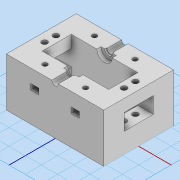
# Autodesk Inventor part: 19_Base_Pezzo_Unico
Saved by Autodesk Inventor 2020 (Build 240168000, 168)
## iProperties
Created: 2019-10-24
Part Number: 19_Base_Pezzo_Unico
Material: Generico
Document SubType Name: Modeling
Designer: socci
Density: 1 g/cm^3
Appearance: Default
Author: socci
Autodesk Inventor part; units mm, degrees
ref_plane "YZ Plane" through (0, 0, 0) normal (1, 0, 0) x (0, 1, 0)
ref_plane "XZ Plane" through (0, 0, 0) normal (0, 1, 0) x (-1, 0, 0)
ref_plane "XY Plane" through (0, 0, 0) normal (0, 0, 1) x (1, 0, 0)
sketch "Schizzo1" plane through (0, 0, 0) normal (0, 1, 0) x (-1, 0, 0)
  line L0 (60, 43) -> (-60, 43)
  line L1 (-60, 43) -> (-60, -43)
  line L2 (-60, -43) -> (60, -43)
  line L3 (60, -43) -> (60, 43)
  line L4 (60, 43) -> (-60, -43) construction
  line L5 (-60, 43) -> (60, -43) construction
  point P0 (0, 0)
  point P1 (0, 0)
  point P2 (0, 0)
  dimension "d0" = 120
  dimension "d1" = 86
  constraints: 12 end point, 3 midpoint, 2 parallel, 1 coincident, 1 horizontal, 1 perpendicular
  measures "d0" distance of L0.start L0.end
  measures "d1" distance of L2.end L0.start
extrude "Estrusione1" add sketch "Schizzo1" along normal blind 60
sketch "Schizzo2" plane through (60, 0, 43) normal (1, 0, 0) x (0, 0, -1)
  line L0 (43, 0) -> (43, 15)
  line L1 (25, 45) -> (61, 45)
  line L2 (61, 45) -> (61, 15)
  line L3 (61, 15) -> (25, 15)
  line L4 (25, 15) -> (25, 45)
  line L5 (25, 45) -> (61, 15) construction
  line L6 (61, 45) -> (25, 15) construction
  point P0 (43, 30)
  dimension "d4" = 15
  dimension "d5" = 36
  dimension "d6" = 30
  constraints: 14 end point, 3 midpoint, 2 parallel, 1 horizontal, 1 perpendicular, 1 vertical
  measures "d4" distance of L0.end L0.start
  measures "d5" distance of L1.start L1.end
  measures "d6" distance of L3.end L1.start
extrude "Estrusione2" cut sketch "Schizzo2" against normal blind 120
sketch "Schizzo3" plane through (60, 15, -18) normal (0, 0, 1) x (1, 0, 0)
  circle A0 centre (-60, 45) radius 9.5
  line L0 (0, 45) -> (-120, 45) projected
  point P0 (-60, -15)
  dimension "d9" = 19
  constraints: 1 centre point, 1 coincident, 1 midpoint
  measures "d9" diameter of A0
extrude "Estrusione3" cut sketch "Schizzo3" against normal blind 5
sketch "Schizzo4" plane through (60, 15, -23) normal (0, 0, 1) x (1, 0, 0)
  circle A0 centre (-60, 45) radius 4
  line L0 (0, 45) -> (-120, 45) projected
  point P0 (-60, -15)
  dimension "d12" = 8
  constraints: 1 centre point, 1 coincident, 1 midpoint
  measures "d12" diameter of A0
extrude "Estrusione4" cut sketch "Schizzo4" against normal blind 20
sketch "Schizzo5" plane through (60, 15, 18) normal (0, 0, -1) x (-1, 0, 0)
  circle A0 centre (60, 45) radius 9.5
  line L0 (120, 45) -> (0, 45) projected
  point P0 (60, -15)
  dimension "d15" = 19
  constraints: 1 centre point, 1 coincident, 1 midpoint
  measures "d15" diameter of A0
extrude "Estrusione5" cut sketch "Schizzo5" against normal blind 5
sketch "Schizzo6" plane through (60, 15, 23) normal (0, 0, -1) x (-1, 0, 0)
  circle A0 centre (60, 45) radius 4
  line L0 (50.5, 45) -> (69.5, 45) projected
  point P0 (60, -15)
  constraints: 1 centre point, 1 coincident, 1 midpoint
extrude "Estrusione6" cut sketch "Schizzo6" against normal blind 20
sketch "Schizzo7" plane through (0, 60, 0) normal (0, 1, 0) x (1, 0, 0)
  line L0 (-4, 43) -> (4, 43) projected
  line L1 (0, 43) -> (0, 18)
  line L2 (60, 18) -> (-60, 18) projected
  line L3 (0, -18) -> (0, -43)
  line L4 (4, -43) -> (-4, -43) projected
  line L5 (-133, 18) -> (-97, 18) construction
  line L6 (-25, 30.5) -> (25, 30.5)
  line L7 (-25, -30.5) -> (25, -30.5)
  point P0 (0, 0)
  point P1 (0, 30.5)
  point P2 (0, -30.5)
  point P3 (-50, 18)
  dimension "d22" = 50
  dimension "d23" = 50
  constraints: 10 end point, 7 midpoint, 2 perpendicular, 1 horizontal
  measures "d22" distance of L6.start L6.end
  measures "d23" distance of L7.start L7.end
hole "Foro1" at (-25, 60, -30.5) at (-25, 60, 30.5) at (25, 60, 30.5) at (25, 60, -30.5) direction (0, -1, 0) diameter 5.9 depth 35 tip angle 118 clearance for "Vite a testa esagonale" size "M5" standard "ANSI - Profilo M Metrico"
sketch "Schizzo8" plane through (-60, 0, 43) normal (0, 0, 1) x (1, 0, 0)
  line L0 (32.05, 60) -> (37.95, 60) projected
  line L1 (82.05, 60) -> (87.95, 60) projected
  line L2 (85, 60) -> (85, 40)
  line L3 (85, 60) -> (65, 60) construction
  line L4 (35, 60) -> (35, 40)
  line L5 (35, 60) -> (15, 60) construction
  line L6 (30, 43.5) -> (40, 43.5)
  line L7 (40, 43.5) -> (40, 36.5)
  line L8 (40, 36.5) -> (30, 36.5)
  line L9 (30, 36.5) -> (30, 43.5)
  line L10 (30, 43.5) -> (40, 36.5) construction
  line L11 (40, 43.5) -> (30, 36.5) construction
  line L12 (80, 43.5) -> (90, 43.5)
  line L13 (90, 43.5) -> (90, 36.5)
  line L14 (90, 36.5) -> (80, 36.5)
  line L15 (80, 36.5) -> (80, 43.5)
  line L16 (80, 43.5) -> (90, 36.5) construction
  line L17 (90, 43.5) -> (80, 36.5) construction
  point P0 (60, 0)
  point P1 (35, 40)
  dimension "d31" = 90
  dimension "d32" = 270
  dimension "d33" = 20
  dimension "d34" = 20
  dimension "d35" = 7
  dimension "d36" = 7
  dimension "d37" = 10
  dimension "d38" = 10
  constraints: 32 end point, 8 midpoint, 4 horizontal, 4 parallel, 4 perpendicular
  measures "d31" angle of L2 L3
  measures "d33" distance of L4.end L4.start
  measures "d34" distance of L2.end L2.start
  measures "d35" distance of L8.end L6.start
  measures "d36" distance of L12.end L13.end
  measures "d37" distance of L7.end L8.end
  measures "d38" distance of L13.end L14.end
extrude "Estrusione7" cut sketch "Schizzo8" against normal blind 19
sketch "Schizzo10" plane through (60, 0, -43) normal (0, 0, -1) x (-1, 0, 0)
  line L0 (85, 60) -> (85, 40)
  line L1 (85, 60) -> (65, 60) construction
  line L2 (35, 60) -> (35, 40)
  line L3 (35, 60) -> (15, 60) construction
  line L4 (30, 43.5) -> (40, 43.5)
  line L5 (40, 43.5) -> (40, 36.5)
  line L6 (40, 36.5) -> (30, 36.5)
  line L7 (30, 36.5) -> (30, 43.5)
  line L8 (30, 43.5) -> (40, 36.5) construction
  line L9 (40, 43.5) -> (30, 36.5) construction
  line L10 (80, 43.5) -> (90, 43.5)
  line L11 (90, 43.5) -> (90, 36.5)
  line L12 (90, 36.5) -> (80, 36.5)
  line L13 (80, 36.5) -> (80, 43.5)
  line L14 (80, 43.5) -> (90, 36.5) construction
  line L15 (90, 43.5) -> (80, 36.5) construction
  line L16 (32.05, 60) -> (37.95, 60) projected
  line L17 (82.05, 60) -> (87.95, 60) projected
  point P0 (60, 0)
  point P1 (50, 0)
  point P2 (35, 40)
  dimension "d42" = 90
  dimension "d43" = 270
  dimension "d44" = 20
  dimension "d45" = 20
  dimension "d46" = 7
  dimension "d47" = 7
  dimension "d48" = 10
  dimension "d49" = 10
  constraints: 32 end point, 8 midpoint, 4 horizontal, 4 parallel, 4 perpendicular
  measures "d42" angle of L0 L1
  measures "d44" distance of L2.start L2.end
  measures "d45" distance of L0.start L0.end
  measures "d46" distance of L6.end L4.start
  measures "d47" distance of L10.end L11.end
  measures "d48" distance of L5.end L6.end
  measures "d49" distance of L11.end L12.end
extrude "Estrusione8" cut sketch "Schizzo10" against normal blind 19
sketch "Schizzo11" plane through (60, 15, 18) normal (0, 0, -1) x (-1, 0, 0)
  line L0 (30.0078, 67.5) -> (89.9922, 22.5) construction
  line L1 (90.0057, 68) -> (30.1859, 18.1994) construction
  line L2 (56, 45) -> (0, 45) projected
  line L3 (120, 45) -> (64, 45) projected
  line L4 (0, 45) -> (120, 45)
  line L5 (60, 45) -> (290, 45) construction
  line L6 (60, 45) -> (60, 19)
  line L7 (60, 45) -> (86, 45) construction
  line L8 (60, 19) -> (92.5948, 19) construction
  line L9 (60, 19) -> (90, 19)
  line L10 (60, 19) -> (90, 19) construction
  line L11 (60, 19) -> (30, 19)
  line L12 (32.05, 10) -> (32.05, 21.5) projected
  line L13 (60, 19) -> (90, 19) construction
  line L14 (60, 45) -> (60, 68)
  line L15 (60, 68) -> (90.0057, 68)
  line L16 (90.0057, 68) -> (30, 68)
  line L17 (30, 68) -> (30, 19)
  line L18 (30, 19) -> (90.0057, 19)
  line L19 (90.0057, 19) -> (90.0057, 68)
  circle A0 centre (60, 45) radius 39.7032
  point P0 (60, -15)
  point P1 (61.2511, 44.0615)
  dimension "d52" = 60
  dimension "d53" = 45.5
  dimension "d72" = 26
  dimension "d73" = 90
  dimension "d75" = 30
  dimension "d76" = 0
  dimension "d77" = 30
  dimension "d78" = 180
  dimension "d79" = 23
  constraints: 34 end point, 8 horizontal, 3 equal length, 3 perpendicular, 2 coincident, 2 midpoint, 2 parallel, 2 point on line, 1 collinear, 3 other
  measures "d52" distance of L0.start L1.start
  measures "d53" distance of L1.start L0.end
  measures "d72" distance of L5.start L6.end
  measures "d73" angle of L6 L7
  measures "d75" distance of L6.end L9.end
  measures "d76" distance between parallel lines of L9 L10
  measures "d77" distance of L6.end L11.end
  measures "d78" angle of L11 L13
  measures "d79" distance of L5.start L14.end
sketch "Schizzo12" plane through (60, 15, 18) normal (0, 0, -1) x (-1, 0, 0)
  line L0 (120, -15) -> (120, 45) projected
  line L1 (120, 45) -> (120, 32)
  line L2 (120, 45) -> (133, 45) construction
  line L3 (120, 32) -> (150, 32)
  line L4 (150, 32) -> (150, 35)
  line L5 (61.2511, 44.0615) -> (261.2511, 44.0615) construction
  arc A0 (56, 45) -> (64, 45) centre (60, 45) ccw projected
  line L6 (60, 45) -> (233.2051, 145)
  line L7 (60, 45) -> (260, 45) construction
  line L8 (150, 35) -> (350, 35) construction
  line L9 (155, 82.5278) -> (145, 99.8483)
  line L10 (150, 35) -> (206.188, 35) construction
  line L11 (155, 82.5278) -> (138, 72.7128)
  line L12 (150, 32) -> (150, 79.641)
  line L13 (150, 79.641) -> (150, 32)
  circle A1 centre (150, 76.1769) radius 3
  line L14 (150, 32) -> (150, 76.1769)
  line L15 (150, 32) -> (120, 10)
  point P0 (60, -15)
  point P1 (61.2511, 44.0615)
  point P2 (61.2511, 44.0615)
  dimension "d54" = 13
  dimension "d55" = 90
  dimension "d56" = 30
  dimension "d57" = 90
  dimension "d58" = 3
  dimension "d61" = 200
  dimension "d62" = 30
  dimension "d66" = 20
  dimension "d67" = 47.641
  dimension "d68" = 6
  dimension "d69" = 44.1769
  constraints: 28 end point, 4 horizontal, 3 point on line, 2 equal length, 2 perpendicular, 2 vertical, 1 centre point, 1 coincident, 1 collinear, 1 parallel, 1 tangent, 3 other
  measures "d54" distance of L0.end L1.end
  measures "d55" angle of L1 L2
  measures "d56" distance of L1.end L3.end
  measures "d57" angle of L3 L1
  measures "d58" distance of L3.end L4.end
  measures "d61" distance of L6.start L6.end
  measures "d62" angle of L7 L6
  measures "d66" distance of L9.start L9.end
  measures "d67" distance of L3.end L12.end
  measures "d68" diameter of A1
  measures "d69" distance of L3.end L14.end
sketch "Schizzo13" plane through (0, 60, 0) normal (0, 1, 0) x (1, 0, 0)
  line L0 (-41, -18) -> (41, -18)
  line L1 (41, -18) -> (41, 18)
  line L2 (41, 18) -> (-41, 18)
  line L3 (-41, 18) -> (-41, -18)
  line L4 (-41, -18) -> (41, 18) construction
  line L5 (41, -18) -> (-41, 18) construction
  point P0 (0, 0)
  point P1 (0, 0)
  point P2 (0, 0)
  dimension "d132" = 82
  dimension "d133" = 36
  constraints: 12 end point, 3 midpoint, 2 parallel, 1 coincident, 1 horizontal, 1 perpendicular
  measures "d132" distance of L1.end L2.end
  measures "d133" distance of L0.end L1.end
extrude "Estrusione9" cut sketch "Schizzo13" against normal blind 20
sketch "Schizzo16" plane through (60, 15, -23) normal (0, 0, 1) x (1, 0, 0)
  circle A0 centre (-60, 45) radius 5
  arc A1 (-64, 45) -> (-56, 45) centre (-60, 45) ccw projected
  point P0 (-60, -15)
  dimension "d94" = 10
  constraints: 1 centre point, 1 coincident
  measures "d94" diameter of A0
extrude "Estrusione11" cut sketch "Schizzo16" against normal blind 2
sketch "Schizzo17" plane through (60, 15, 23) normal (0, 0, -1) x (-1, 0, 0)
  arc A0 (56, 45) -> (64, 45) centre (60, 45) ccw projected
  circle A1 centre (60, 45) radius 5
  point P0 (60, -15)
  dimension "d97" = 10
  constraints: 1 centre point, 1 coincident
  measures "d97" diameter of A1
extrude "Estrusione12" cut sketch "Schizzo17" against normal blind 2
sketch "Schizzo21" plane through (60, 15, 18) normal (0, 1, 0) x (1, 0, 0)
  line L0 (-19, 36) -> (-19, 0) projected
  line L1 (-101, 0) -> (-101, 36) projected
  line L2 (-19, 0) -> (-50.5, 0) projected
  line L3 (-50.5, 36) -> (-19, 36) projected
  line L4 (-101, 36) -> (-69.5, 36) projected
  line L5 (-69.5, 0) -> (-101, 0) projected
  line L6 (-19, 36) -> (-19, 0)
  line L7 (-19, 0) -> (0, 0)
  line L8 (0, 0) -> (0, 36)
  line L9 (0, 36) -> (-19, 36)
  line L10 (-101, 36) -> (-101, 0)
  line L11 (-101, 0) -> (-120, 0)
  line L12 (-120, 0) -> (-120, 36)
  line L13 (-120, 36) -> (-101, 36)
  line L14 (-120, 61) -> (-120, -25) projected
  line L15 (0, -25) -> (0, 61) projected
  point P0 (-60, 18)
  constraints: 16 end point, 5 equal length, 3 perpendicular, 2 collinear
extrude "Estrusione14" add sketch "Schizzo21" along normal blind 10
sketch "Schizzo15" plane through (0, 60, 0) normal (0, 1, 0) x (1, 0, 0)
  line L0 (-60, 43) -> (-60, -43) projected
  line L1 (60, -43) -> (60, 43) projected
  line L2 (60, 0) -> (66, 0) construction
  line L3 (-60, -18) -> (-60, 18) projected
  line L4 (-49, 0) -> (-42, 0) construction
  line L5 (-49, 0) -> (-42, 0) construction
  line L6 (-43, 0) -> (-49, 0)
  line L7 (43, 0) -> (49, 0)
  line L8 (43, 0) -> (49, 0) construction
  line L9 (-49, 0) -> (-49, 7)
  line L10 (-49, 0) -> (-42, 0) construction
  line L11 (-49, 0) -> (-49, -7)
  line L12 (-49, 0) -> (-42, 0) construction
  line L13 (49, 0) -> (49, 7)
  line L14 (49, 0) -> (56, 0) construction
  line L15 (49, 0) -> (49, -7)
  line L16 (49, 0) -> (56, 0) construction
  point P0 (0, 0)
  dimension "d134" = 6
  dimension "d137" = 6
  dimension "d138" = 0
  dimension "d139" = 7
  dimension "d140" = 90
  dimension "d141" = 7
  dimension "d142" = 90
  dimension "d143" = 7
  dimension "d144" = 90
  dimension "d145" = 7
  dimension "d146" = 90
  constraints: 28 end point, 10 horizontal, 7 coincident, 5 equal length, 3 vertical, 1 midpoint, 1 perpendicular
  measures "d134" distance of L6.start L6.end
  measures "d137" distance of L7.start L7.end
  measures "d138" distance between parallel lines of L7 L8
  measures "d139" distance of L9.start L9.end
  measures "d140" angle of L10 L9
  measures "d141" distance of L9.start L11.end
  measures "d142" angle of L11 L12
  measures "d143" distance of L13.start L13.end
  measures "d144" angle of L14 L13
  measures "d145" distance of L13.start L15.end
  measures "d146" angle of L15 L16
hole "Foro5" at (49, 60, 7) at (49, 60, -7) at (-49, 60, 7) at (-49, 60, -7) direction (0, -1, 0) diameter 7 depth 60 tip angle 118 clearance for "Vite a testa piana" size "M6" standard "ANSI - Profilo M Metrico"
sketch "Schizzo22" plane through (0, 0, 0) normal (0, -1, 0) x (1, 0, 0)
  circle A0 centre (-49, -7) radius 3.5 projected
  circle A1 centre (-49, 7) radius 3.5 projected
  circle A2 centre (49, -7) radius 3.5 projected
  circle A3 centre (49, 7) radius 3.5 projected
  circle A4 centre (-49, -7) radius 5.5
  circle A5 centre (-49, 7) radius 5.5
  circle A6 centre (49, -7) radius 5.5
  circle A7 centre (49, 7) radius 5.5
  line L0 (52.1754, -1.5) -> (55.3509, -7)
  line L1 (55.3509, -7) -> (52.1754, -12.5)
  line L2 (52.1754, -12.5) -> (45.8246, -12.5)
  line L3 (45.8246, -12.5) -> (42.6491, -7)
  line L4 (42.6491, -7) -> (45.8246, -1.5)
  line L5 (45.8246, -1.5) -> (52.1754, -1.5)
  line L6 (45.8246, 1.5) -> (42.6491, 7)
  line L7 (42.6491, 7) -> (45.8246, 12.5)
  line L8 (45.8246, 12.5) -> (52.1754, 12.5)
  line L9 (52.1754, 12.5) -> (55.3509, 7)
  line L10 (55.3509, 7) -> (52.1754, 1.5)
  line L11 (52.1754, 1.5) -> (45.8246, 1.5)
  line L12 (-45.8246, -1.5) -> (-42.6491, -7)
  line L13 (-42.6491, -7) -> (-45.8246, -12.5)
  line L14 (-45.8246, -12.5) -> (-52.1754, -12.5)
  line L15 (-52.1754, -12.5) -> (-55.3509, -7)
  line L16 (-55.3509, -7) -> (-52.1754, -1.5)
  line L17 (-52.1754, -1.5) -> (-45.8246, -1.5)
  line L18 (-52.1754, 1.5) -> (-55.3509, 7)
  line L19 (-55.3509, 7) -> (-52.1754, 12.5)
  line L20 (-52.1754, 12.5) -> (-45.8246, 12.5)
  line L21 (-45.8246, 12.5) -> (-42.6491, 7)
  line L22 (-42.6491, 7) -> (-45.8246, 1.5)
  line L23 (-45.8246, 1.5) -> (-52.1754, 1.5)
  point P0 (0, 0)
  point P1 (49, -1.5)
  point P2 (49, 1.5)
  point P3 (-49, -1.5)
  point P4 (-49, 1.5)
  dimension "d167" = 11
  dimension "d168" = 11
  dimension "d169" = 11
  dimension "d170" = 11
  constraints: 48 end point, 8 coincident, 4 midpoint, 4 vertical alignment, 2 point on line, 60 other
extrude "Estrusione15" cut sketch "Schizzo22" against normal blind 7 contours A0 | A1 | A2 | A3 | A4 | A4 L12 L13 | A4 L17 L12 | L13 L14 A4 | A4 L16 L17 | L14 L15 A4 | A4 L15 L16 | A5 | A5 L21 L22 | A5 L20 L21 | L22 L23 A5 | A5 L19 L20 | L23 L18 A5 | A5 L18 L19 | A6 | A6 L0 L1 | A6 L5 L0 | L1 L2 A6 | A6 L4 L5 | L2 L3 A6 | A6 L3 L4 | A7 | A7 L9 L10 | A7 L8 L9 | L10 L11 A7 | A7 L7 L8 | L11 L6 A7 | A7 L6 L7
